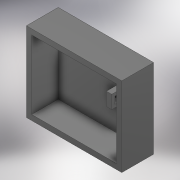
# Autodesk Inventor part: Wasserbecken
Saved by Autodesk Inventor 2020 (Build 240168000, 168)
## iProperties
Created: 2022-02-20
Part Number: Wasserbecken
Material: Acetalharz, Schwarz
Document SubType Name: Modeling
Designer: Julian Uhl
Density: 1.425 g/cm^3
Appearance: Glatt - Schwarz
Mass: 103.858 g
Surface Area: 310.28 cm^2
Volume: 72.8825 cm^3
Author: Julian Uhl
Autodesk Inventor part; units mm, degrees
ref_plane "YZ Plane" through (0, 0, 0) normal (1, 0, 0) x (0, 1, 0)
ref_plane "XZ Plane" through (0, 0, 0) normal (0, 1, 0) x (-1, 0, 0)
ref_plane "XY Plane" through (0, 0, 0) normal (0, 0, 1) x (1, 0, 0)
sketch "Skizze1" plane through (0, 0, 0) normal (0, 0, 1) x (1, 0, 0)
  line L0 (-18, 0) -> (108, 0) projected
  line L1 (0, -15) -> (0, 90) projected
  line L2 (0, 0) -> (90, 0)
  line L3 (90, 0) -> (90, 75)
  line L4 (90, 75) -> (0, 75)
  line L5 (0, 75) -> (0, 0)
  line L6 (5, 70) -> (85, 70)
  line L7 (85, 70) -> (85, 5)
  line L8 (85, 5) -> (5, 5)
  line L9 (5, 5) -> (5, 70)
  point P0 (0, 75)
  dimension "d0" = 75
  dimension "d1" = 90
  dimension "d2" = 5
  dimension "d3" = 5
  dimension "d4" = 5
  dimension "d5" = 5
  constraints: 16 end point, 4 parallel, 2 horizontal, 2 perpendicular
  measures "d0" distance between parallel lines of L0 L4
  measures "d1" distance between parallel lines of L3 L1
  measures "d2" distance between parallel lines of L4 L6
  measures "d3" distance between parallel lines of L5 L9
  measures "d4" distance between parallel lines of L2 L8
  measures "d5" distance between parallel lines of L3 L7
extrude "Extrusion1" add sketch "Skizze1" along normal blind 25
sketch "Skizze2" plane through (0, 0, 0) normal (0, 0, -1) x (-1, 0, 0)
  line L0 (0, 75) -> (0, 0) projected
  line L1 (0, 75) -> (-90, 75)
  line L2 (-90, 75) -> (-90, 0)
  line L3 (-90, 0) -> (0, 0)
  line L4 (0, 0) -> (0, 75)
  constraints: 8 end point, 2 parallel, 1 horizontal, 1 perpendicular
extrude "Extrusion2" add sketch "Skizze2" along normal blind 5
sketch "Skizze3" plane through (0, 0, 0) normal (0, 0, 1) x (1, 0, 0)
  line L0 (60, 31.25) -> (65, 31.25)
  line L1 (65, 31.25) -> (65, 43.75)
  line L2 (65, 43.75) -> (60, 43.75)
  line L3 (60, 43.75) -> (60, 31.25)
  line L4 (85, 5) -> (5, 5) projected
  line L5 (5, 5) -> (5, 70) projected
  point P0 (0, 0)
  dimension "d10" = 12.5
  dimension "d11" = 5
  dimension "d12" = 26.25
  dimension "d13" = 55
  constraints: 8 end point, 2 parallel, 1 horizontal, 1 perpendicular
  measures "d10" distance between parallel lines of L2 L0
  measures "d11" distance between parallel lines of L3 L1
  measures "d12" distance between parallel lines of L4 L0
  measures "d13" distance between parallel lines of L5 L3
extrude "Extrusion3" add sketch "Skizze3" along normal blind 9.5
sketch "Skizze4" plane through (60, 31.25, 0) normal (-1, 0, 0) x (0, 0, 1)
  line L0 (0, 12.5) -> (0, 0) projected
  line L1 (0, 3) -> (6.5, 3)
  line L2 (6.5, 3) -> (6.5, 9.5)
  line L3 (6.5, 9.5) -> (0, 9.5)
  line L4 (0, 9.5) -> (0, 3)
  line L5 (0, 0) -> (9.5, 0) projected
  point P0 (0, -31.25)
  point P1 (0, 9.5)
  dimension "d16" = 6.5
  dimension "d17" = 6.5
  dimension "d18" = 3
  constraints: 8 end point, 2 parallel, 1 horizontal, 1 perpendicular, 1 point on line
  measures "d16" distance of L1.end L2.end
  measures "d17" distance between parallel lines of L2 L0
  measures "d18" distance between parallel lines of L5 L1
extrude "Extrusion4" cut sketch "Skizze4" against normal blind 5
